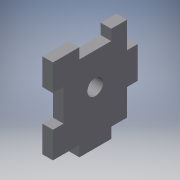
# Autodesk Inventor part: Part2
Saved by Autodesk Inventor 2018 (Build 220112000, 112)
## iProperties
Created: 2018-05-22
Part Number: Part2
Material: Generic
Document SubType Name: Modeling
Designer: Administrator
Density: 1 g/cm^3
Appearance: Default
Author: Administrator
Autodesk Inventor part; units mm, degrees
ref_plane "YZ Plane" through (0, 0, 0) normal (1, 0, 0) x (0, 1, 0)
ref_plane "XZ Plane" through (0, 0, 0) normal (0, 1, 0) x (-1, 0, 0)
ref_plane "XY Plane" through (0, 0, 0) normal (0, 0, 1) x (1, 0, 0)
sketch "Sketch1" plane through (0, 0, 0) normal (1, 0, 0) x (0, 1, 0)
  line L0 (1.6542, 74.5762) -> (-23.7458, 74.5762)
  line L1 (-23.7458, 74.5762) -> (-23.7458, 49.1762)
  line L2 (-23.7458, 49.1762) -> (1.6542, 49.1762)
  line L3 (1.6542, 49.1762) -> (1.6542, 74.5762)
  line L4 (-23.7458, 66.6387) -> (-26.9208, 66.6387)
  line L5 (-26.9208, 66.6387) -> (-26.9208, 57.1137)
  line L6 (-26.9208, 57.1137) -> (-23.7458, 57.1137)
  line L7 (-23.7458, 57.1137) -> (-23.7458, 66.6387)
  point P0 (0, 0)
  dimension "d0" = 25.4
  dimension "d1" = 25.4
  dimension "d4" = 3.175
  dimension "d5" = 7.9375
  dimension "d6" = 7.9375
  constraints: 16 end point, 4 parallel, 2 horizontal, 2 perpendicular, 1 point on line
  measures "d0" distance between parallel lines of L2 L0
  measures "d1" distance between parallel lines of L3 L1
  measures "d4" distance between parallel lines of L1 L5
  measures "d5" distance between parallel lines of L2 L6
  measures "d6" distance between parallel lines of L0 L4
extrude "Extrusion2" add sketch "Sketch1" along normal blind 3.175
sketch "Sketch2" plane through (3.175, 0, 0) normal (1, 0, 0) x (0, 0, -1)
  line L0 (-74.5762, 1.6542) -> (-74.5762, -23.7458) projected
  line L1 (-74.5762, -6.2833) -> (-71.4012, -6.2833)
  line L2 (-71.4012, -6.2833) -> (-71.4012, -15.8083)
  line L3 (-71.4012, -15.8083) -> (-74.5762, -15.8083)
  line L4 (-74.5762, -15.8083) -> (-74.5762, -6.2833)
  line L5 (-74.5762, -23.7458) -> (-66.6387, -23.7458) projected
  line L6 (-49.1762, 1.6542) -> (-74.5762, 1.6542) projected
  line L7 (-49.1762, 1.6542) -> (-74.5762, 1.6542) projected
  line L8 (-49.1762, -23.7458) -> (-49.1762, 1.6542) projected
  line L9 (-52.3512, 1.6542) -> (-49.1762, 1.6542)
  line L10 (-49.1762, 1.6542) -> (-49.1762, -6.2833)
  line L11 (-49.1762, -6.2833) -> (-52.3512, -6.2833)
  line L12 (-52.3512, -6.2833) -> (-52.3512, 1.6542)
  line L13 (-57.1137, -23.7458) -> (-49.1762, -23.7458) projected
  line L14 (-49.1762, -23.7458) -> (-52.3512, -23.7458)
  line L15 (-52.3512, -23.7458) -> (-52.3512, -15.8083)
  line L16 (-52.3512, -15.8083) -> (-49.1762, -15.8083)
  line L17 (-49.1762, -15.8083) -> (-49.1762, -23.7458)
  line L18 (-66.6387, 1.6542) -> (-57.1137, 1.6542)
  line L19 (-57.1137, 1.6542) -> (-57.1137, -1.5208)
  line L20 (-57.1137, -1.5208) -> (-66.6387, -1.5208)
  line L21 (-66.6387, -1.5208) -> (-66.6387, 1.6542)
  point P0 (0, 0)
  dimension "d9" = 3.175
  dimension "d10" = 7.9375
  dimension "d11" = 7.9375
  dimension "d23" = 3.175
  dimension "d24" = 7.9375
  dimension "d25" = 7.9375
  dimension "d28" = 3.175
  dimension "d29" = 3.175
  constraints: 32 end point, 8 parallel, 5 point on line, 4 horizontal, 4 perpendicular
  measures "d9" distance between parallel lines of L2 L0
  measures "d10" distance between parallel lines of L5 L3
  measures "d11" distance between parallel lines of L6 L1
  measures "d23" distance between parallel lines of L6 L20
  measures "d24" distance between parallel lines of L8 L19
  measures "d25" distance between parallel lines of L0 L21
  measures "d28" distance between parallel lines of L10 L12
  measures "d29" distance between parallel lines of L8 L15
sketch "Sketch3" plane through (3.175, 0, 0) normal (1, 0, 0) x (0, 0, -1)
  line L0 (-49.1762, 1.6542) -> (-74.5762, 1.6542) projected
  line L1 (-74.5762, 1.6542) -> (-74.5762, -23.7458) projected
  point P0 (0, 0)
  point P1 (-61.8762, -11.0458)
  point P2 (-51.892, 1.6542)
  point P3 (-74.5762, -6.2833)
  dimension "d14" = 12.7
  dimension "d15" = 12.7
  measures "d14" distance from line of L0 point (-61.876, -11.046)
  measures "d15" distance from line of L1 point (-61.876, -11.046)
hole "Hole1" at (3.175, -11.0458, 61.8762) direction (-1, 0, 0) diameter 4.7625 depth 3.175 tip angle 118
extrude "Extrusion4" cut sketch "Sketch2" against normal blind 3.175
body "Solid2"
